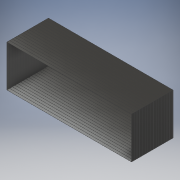
# Autodesk Inventor part: Pool
Saved by Autodesk Inventor 2019 (Build 230136000, 136)
## iProperties
Created: 2021-05-11
Part Number: Pool
Material: Steel, Galvanized
Document SubType Name: Modeling
Designer: jamieson-bl
Density: 7.85 g/cm^3
Appearance: Galvanized
Mass: 3.50982e+06 g
Surface Area: 486812 cm^2
Volume: 2.95439e+06 cm^3
Author: jamieson-bl
Autodesk Inventor part; units mm, degrees
ref_plane "YZ Plane" through (0, 0, 0) normal (1, 0, 0) x (0, 1, 0)
ref_plane "XZ Plane" through (0, 0, 0) normal (0, 1, 0) x (-1, 0, 0)
ref_plane "XY Plane" through (0, 0, 0) normal (0, 0, 1) x (1, 0, 0)
sketch "Sketch1" plane through (0, 0, 0) normal (0, 0, 1) x (1, 0, 0)
  line L0 (2286, -762) -> (-2286, -762)
  line L1 (-2286, -762) -> (-2286, 762)
  line L2 (-2286, 762) -> (2286, 762)
  line L3 (2286, 762) -> (2286, -762)
  line L4 (2286, -762) -> (-2286, 762) construction
  line L5 (-2286, -762) -> (2286, 762) construction
  point P0 (0, 0)
  dimension "d0" = 4572
  dimension "d1" = 1524
  constraints: 12 end point, 2 midpoint, 2 parallel, 1 horizontal, 1 perpendicular
  measures "d0" distance of L1.end L2.end
  measures "d1" distance of L0.end L1.end
extrude "Extrusion1" add sketch "Sketch1" along normal blind 1524
sketch "Sketch2" plane through (0, 0, 1524) normal (0, 0, 1) x (1, 0, 0)
  line L0 (2283.26, -759.26) -> (-2283.26, -759.26)
  line L1 (-2283.26, -759.26) -> (-2283.26, 759.26)
  line L2 (-2283.26, 759.26) -> (2283.26, 759.26)
  line L3 (2283.26, 759.26) -> (2283.26, -759.26)
  line L4 (2283.26, -759.26) -> (-2283.26, 759.26) construction
  line L5 (-2283.26, -759.26) -> (2283.26, 759.26) construction
  line L6 (-2286, -762) -> (2286, -762) projected
  line L7 (2286, 762) -> (-2286, 762) projected
  line L8 (-2286, 762) -> (-2286, -762) projected
  line L9 (2286, -762) -> (2286, 762) projected
  point P0 (0, 0)
  dimension "d4" = 4566.52
  dimension "d5" = 1518.52
  dimension "d8" = 2.74
  dimension "d9" = 2.74
  dimension "d10" = 4572
  dimension "d11" = 2.74
  dimension "d12" = 2.74
  constraints: 12 end point, 2 midpoint, 2 parallel, 1 horizontal, 1 perpendicular
  measures "d4" distance of L1.end L2.end
  measures "d5" distance of L0.end L1.end
  measures "d8" distance between parallel lines of L6 L0
  measures "d9" distance between parallel lines of L7 L2
  measures "d10" distance of L6.start L6.end
  measures "d11" distance between parallel lines of L8 L1
  measures "d12" distance between parallel lines of L9 L3
extrude "Extrusion2" cut sketch "Sketch2" against normal blind 1521.26 contours L0 L1 L2 L3
sketch "Sketch4" plane through (0, 0, 0) normal (1, 0, 0) x (0, 1, 0)
  line L0 (-762, 1524) -> (762, 1524) projected
  line L1 (-762, 1524) -> (762, 1524)
  line L2 (-762, 1524) -> (762, 1524)
  line L3 (762, 1524) -> (762, 1424)
  line L4 (762, 0) -> (762, 1524) projected
  line L5 (762, 1424) -> (-762, 1424)
  line L6 (-762, 1424) -> (-762, 1324)
  line L7 (-762, 0) -> (-762, 1524) projected
  line L8 (-762, 1324) -> (762, 1324)
  line L9 (762, 1324) -> (762, 1224)
  line L10 (762, 1224) -> (-762, 1224)
  line L11 (-762, 1224) -> (-762, 1124)
  line L12 (-762, 1124) -> (762, 1124)
  line L13 (762, 1124) -> (762, 1024)
  line L14 (762, 1024) -> (-762, 1024)
  line L15 (-762, 1024) -> (-762, 924)
  line L16 (-762, 924) -> (762, 924)
  line L17 (762, 924) -> (762, 824)
  line L18 (762, 824) -> (-762, 824)
  line L19 (-762, 824) -> (-762, 724)
  line L20 (-762, 724) -> (762, 724)
  line L21 (762, 724) -> (762, 624)
  line L22 (762, 624) -> (-762, 624)
  line L23 (-762, 624) -> (-762, 524)
  line L24 (-762, 524) -> (762, 524)
  line L25 (762, 524) -> (762, 424)
  line L26 (762, 424) -> (-762, 424)
  line L27 (-762, 424) -> (-762, 324)
  line L28 (-762, 324) -> (762, 324)
  line L29 (762, 324) -> (762, 224)
  line L30 (762, 224) -> (-762, 224)
  line L31 (-762, 224) -> (-762, 124)
  line L32 (-762, 124) -> (762, 124)
  line L33 (762, 124) -> (762, 24)
  line L34 (762, 24) -> (-762, 24)
  point P0 (0, 0)
  dimension "d19" = 100
  dimension "d20" = 100
  dimension "d21" = 100
  dimension "d22" = 100
  dimension "d23" = 100
  dimension "d24" = 100
  dimension "d25" = 100
  dimension "d26" = 100
  dimension "d27" = 100
  dimension "d28" = 100
  dimension "d29" = 100
  dimension "d30" = 100
  dimension "d31" = 100
  dimension "d32" = 100
  dimension "d33" = 100
  constraints: 64 end point, 29 point on line, 15 perpendicular, 2 collinear
  measures "d19" distance of L0.end L3.end
  measures "d20" distance of L5.end L6.end
  measures "d21" distance of L8.end L9.end
  measures "d22" distance of L10.end L11.end
  measures "d23" distance of L12.end L13.end
  measures "d24" distance of L14.end L15.end
  measures "d25" distance of L16.end L17.end
  measures "d26" distance of L18.end L19.end
  measures "d27" distance of L20.end L21.end
  measures "d28" distance of L22.end L23.end
  measures "d29" distance of L24.end L25.end
  measures "d30" distance of L26.end L27.end
  measures "d31" distance of L28.end L29.end
  measures "d32" distance of L30.end L31.end
  measures "d33" distance of L32.end L33.end
split_face "Split1"
